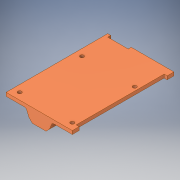
# Autodesk Inventor part: Raspi3B+_Case
Saved by Autodesk Inventor 2018 (Build 220112000, 112)
## iProperties
Created: 2018-06-22
Part Number: Raspi3B+_Case
Material: Generic
Document SubType Name: Modeling
Designer: snipe
Density: 1 g/cm^3
Appearance: Default
Sending System: SolidWorks 2017
Last Author: Dan
Last Saved: 2018-12-13
Author: snipe
Autodesk Inventor part; units mm, degrees
ref_plane "YZ Plane" through (0, 0, 0) normal (1, 0, 0) x (0, 1, 0)
ref_plane "XZ Plane" through (0, 0, 0) normal (0, 1, 0) x (-1, 0, 0)
ref_plane "Work Plane3" through (-25, 0, 42.5) normal (0, -1, 0) x (1, 0, 0)
sketch "Sketch1" plane through (-25, 0, 42.5) normal (0, -1, 0) x (1, 0, 0)
  line L0 (28.4781, -19.558) -> (28.4781, -33.5534) projected
  arc A0 (53, -3) -> (50, 0) centre (50, -3) ccw projected
  line L1 (0, 0) -> (50, 0) projected
  arc A1 (0, 0) -> (-3, -3) centre (0, -3) ccw projected
  line L2 (-3, -82) -> (-3, -3) projected
  arc A2 (-3, -82) -> (0, -85) centre (0, -82) ccw projected
  line L3 (50, -85) -> (0, -85) projected
  arc A3 (50, -85) -> (53, -82) centre (50, -82) ccw projected
  line L4 (53, -3) -> (53, -82) projected
  circle A4 centre (49.5, -61.5) radius 1.75 projected
  circle A5 centre (0.5, -61.5) radius 1.75 projected
  circle A6 centre (0.5, -3.5) radius 1.75 projected
  circle A7 centre (49.5, -3.5) radius 1.75 projected
  line L5 (-3, 0) -> (53, 0)
  line L6 (53, 0) -> (53, -88.9)
  line L7 (53, -88.9) -> (-3, -88.9)
  line L8 (-3, -88.9) -> (-3, 0)
  point P0 (25, -42.5)
  dimension "d0" = 88.9
  constraints: 8 end point, 2 parallel, 1 horizontal, 1 perpendicular, 1 point on line
  measures "d0" distance of L5.end L6.end
extrude "Extrusion1" add sketch "Sketch1" along normal blind 3.175
sketch "Sketch2" plane through (-25, -3.175, 42.5) normal (0, -1, 0) x (1, 0, 0)
  circle A0 centre (49.5, -3.5) radius 1.75 projected
  circle A1 centre (0.5, -3.5) radius 1.75 projected
  circle A2 centre (0.5, -61.5) radius 1.75 projected
  circle A3 centre (49.5, -61.5) radius 1.75 projected
  line L0 (53, 0) -> (-3, 0) projected
  line L1 (-3, 0) -> (-3, -88.9) projected
  line L2 (-3, -88.9) -> (53, -88.9) projected
  line L3 (53, -88.9) -> (53, 0) projected
  line L4 (-3, -88.9) -> (53, -88.9) projected
  line L5 (55.8, 2.8) -> (55.8, -91.7)
  line L6 (-5.8, -91.7) -> (-5.8, 2.8)
  line L7 (53, 0) -> (55.8, 2.8)
  line L8 (53, 0) -> (58.3967, 0) construction
  line L9 (55.8, 2.8) -> (-5.8, 2.8)
  line L10 (53, -88.9) -> (61.5609, -88.9) construction
  line L11 (55.8, -91.7) -> (-5.8, -91.7)
  point P0 (25, -42.5)
  dimension "d3" = 45
  constraints: 14 end point, 4 horizontal, 1 parallel
  measures "d3" angle of L8 L7
extrude "Extrusion2" add sketch "Sketch2" against normal blind 3.175 contours L5 L11 L6 L9
sketch "Sketch3" plane through (-25, 0, 42.5) normal (0, 1, 0) x (1, 0, 0)
  line L0 (-5.8, -2.8) -> (55.8, -2.8) projected
  line L1 (55.8, -2.8) -> (55.8, 91.7) projected
  line L2 (55.8, 91.7) -> (-5.8, 91.7) projected
  line L3 (-5.8, 91.7) -> (-5.8, -2.8) projected
  line L4 (53, 3.55) -> (55.8, 3.55)
  line L5 (55.8, 3.55) -> (55.8, 85.35)
  line L6 (55.8, 85.35) -> (53, 85.35)
  line L7 (53, 85.35) -> (53, 3.55)
  point P0 (25, 42.5)
  dimension "d7" = 6.35
  dimension "d20" = 6.35
  constraints: 8 end point, 2 parallel, 1 horizontal, 1 perpendicular, 1 point on line
  measures "d7" distance between parallel lines of L0 L4
  measures "d20" distance between parallel lines of L2 L6
extrude "Extrusion3" cut sketch "Sketch3" against normal blind 15.875 contours L4 L7 L6 L1
sketch "Sketch5" plane through (-25, 0, 42.5) normal (0, 1, 0) x (1, 0, 0)
  line L0 (-3, 88.9) -> (16.05, 88.9)
  line L1 (16.05, 88.9) -> (16.05, 91.7575)
  line L2 (16.05, 91.7575) -> (-3, 91.7575)
  line L3 (-3, 91.7575) -> (-3, 88.9)
  line L4 (55.8, 3.55) -> (53, 3.55) projected
  line L5 (53, 85.35) -> (55.8, 85.35) projected
  line L6 (55.8, 85.35) -> (55.8, 91.7) projected
  line L7 (55.8, 91.7) -> (-5.8, 91.7) projected
  line L8 (-5.8, 91.7) -> (-5.8, -2.8) projected
  line L9 (-5.8, -2.8) -> (55.8, -2.8) projected
  line L10 (55.8, -2.8) -> (55.8, 3.55) projected
  line L11 (53, 3.55) -> (53, 85.35) projected
  point P0 (25, 42.5)
  dimension "d15" = 19.05
  dimension "d16" = 2.8575
  constraints: 8 end point, 2 parallel, 1 horizontal, 1 perpendicular
  measures "d15" distance of L1.end L2.end
  measures "d16" distance of L2.end L0.start
extrude "Extrusion5" cut sketch "Sketch5" against normal blind 15.875 contours L3 L7 L1 L0 | L3 L2 L1 L7
sketch "Sketch6" plane through (-25, -3.175, 42.5) normal (0, -1, 0) x (1, 0, 0)
  line L0 (16.05, -88.9) -> (16.05, -91.7) projected
  line L1 (16.05, -91.7) -> (55.8, -91.7) projected
  line L2 (55.8, -91.7) -> (55.8, -85.35) projected
  line L3 (55.8, -85.35) -> (53, -85.35) projected
  line L4 (53, -85.35) -> (53, -3.55) projected
  line L5 (53, -3.55) -> (55.8, -3.55) projected
  line L6 (55.8, -3.55) -> (55.8, 2.8) projected
  line L7 (55.8, 2.8) -> (-5.8, 2.8) projected
  line L8 (-5.8, 2.8) -> (-5.8, -91.7) projected
  line L9 (-5.8, -91.7) -> (-3, -91.7) projected
  line L10 (-3, -91.7) -> (-3, -88.9) projected
  line L11 (-3, -88.9) -> (16.05, -88.9) projected
  circle A0 centre (49.5, -61.5) radius 1.75 projected
  circle A1 centre (0.5, -61.5) radius 1.75 projected
  circle A2 centre (0.5, -3.5) radius 1.75 projected
  circle A3 centre (49.5, -3.5) radius 1.75 projected
  line L12 (34.525, 2.8) -> (34.525, -0.0575) projected
  line L13 (16.05, -88.9) -> (-3, -88.9) projected
  line L14 (16.05, -0.0575) -> (15.475, -0.0575)
  line L15 (15.475, -0.0575) -> (15.475, -88.9)
  line L16 (15.475, -88.9) -> (16.05, -88.9)
  line L17 (34.525, -88.9) -> (34.525, -0.0575)
  line L18 (16.05, -91.7) -> (55.8, -91.7) projected
  line L19 (16.05, -88.9) -> (16.05, -91.7)
  line L20 (16.05, -91.7) -> (34.525, -91.7)
  line L21 (34.525, -91.7) -> (34.525, -88.9)
  line L22 (15.475, -0.0575) -> (16.05, -0.0575)
  line L23 (34.525, -0.0575) -> (34.525, 2.8)
  line L24 (34.525, 2.8) -> (15.475, 2.8)
  line L25 (15.475, 2.8) -> (15.475, -0.0575)
  point P0 (25, -42.5)
  constraints: 22 end point, 5 parallel, 2 horizontal, 2 perpendicular, 2 point on line
extrude "Extrusion6" add sketch "Sketch6" along normal blind 9.525 contours L11 L15 L25 L7 L12 L17 L21 L1 L0
chamfer "Chamfer1" distance 3.175 angle 45 2 edges at (-9.525, -3.175, -0.55) (9.525, -3.175, -1.95)
chamfer "Chamfer2" distance 3.175 angle 45 2 edges at (9.525, -6.35, -1.95) (-9.525, -6.35, -0.55)
chamfer "Chamfer3" distance 3.175 angle 45 2 edges at (9.525, -12.7, -1.95) (-9.525, -12.7, -0.55)
fillet "Fillet1" radius 3.175 2 edges at (-12.7, -3.175, -0.55) (12.7, -3.175, -1.95)
body "Solid1"
